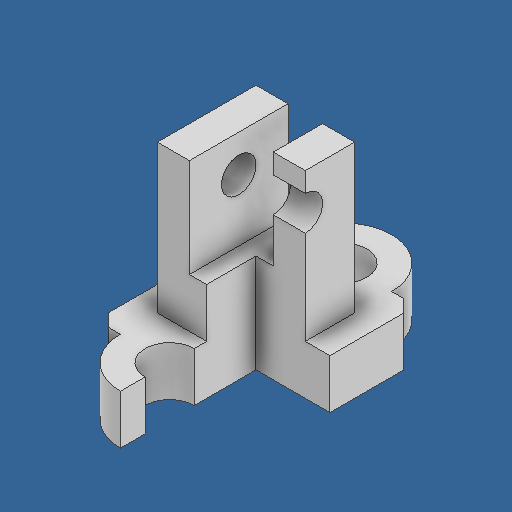
# Autodesk Inventor part: пч2020
Saved by Autodesk Inventor 2025 (Build 290162000, 162)
## iProperties
Created: 2024-12-02
Part Number: пч2020
Material: Типовые
Document SubType Name: Modeling
Designer: Asus
Density: 1 g/cm^3
Appearance: По умолчанию
Author: Asus
Autodesk Inventor part; units mm, degrees
ref_plane "YZ Plane" through (0, 0, 0) normal (1, 0, 0) x (0, 1, 0)
ref_plane "XY Plane" through (0, 0, 0) normal (0, 0, 1) x (1, 0, 0)
sketch "Эскиз1" plane through (0, 0, 0) normal (0, 1, 0) x (-1, 0, 0)
  line L0 (-30, 0) -> (-30, -30)
  line L1 (-30, 0) -> (-30, 30)
  circle A0 centre (0, 35) radius 10
  arc A1 (20, 35) -> (-20, 35) centre (0, 35) ccw
  line L2 (-25, 35) -> (-30, 30)
  circle A2 centre (0, -35) radius 10
  arc A3 (-20, -35) -> (20, -35) centre (0, -35) ccw
  line L3 (-30, -30) -> (-25, -35)
  line L4 (30, 30) -> (30, -30)
  line L5 (25, 35) -> (30, 30)
  line L6 (25, -35) -> (30, -30)
  line L7 (-25, 35) -> (-20, 35)
  line L8 (20, 35) -> (25, 35)
  line L9 (-25, -35) -> (-20, -35)
  line L10 (20, -35) -> (25, -35)
  point P0 (0, 0)
  point P1 (-30, -35)
  point P2 (-30, 35)
  point P3 (30, 35)
  point P4 (30, -35)
  point P5 (30, 35)
  point P6 (30, -35)
  dimension "d0" = 35
  dimension "d1" = 35
  dimension "d2" = 20
  dimension "d3" = 40
  dimension "d4" = 5
  dimension "d5" = 5
  dimension "d6" = 20
  dimension "d7" = 40
  dimension "d8" = 5
  dimension "d9" = 5
  dimension "d10" = 5
  dimension "d11" = 5
  dimension "d12" = 5
  dimension "d13" = 5
  constraints: 22 end point, 8 point on line, 4 centre point, 4 horizontal, 4 point on circle, 2 coincident, 2 perpendicular, 2 vertical
  measures "d0" distance of L0.start point (-30, -35)
  measures "d1" distance of L0.start point (-30, 35)
  measures "d2" diameter of A0
  measures "d3" diameter of A1
  measures "d4" distance of L2.start point (-30, 35)
  measures "d5" distance of L1.end point (-30, 35)
  measures "d6" diameter of A2
  measures "d7" diameter of A3
  measures "d8" distance of L0.end point (-30, -35)
  measures "d9" distance of L3.end point (-30, -35)
  measures "d10" distance of L5.start point (30, 35)
  measures "d11" distance of L4.start point (30, 35)
  measures "d12" distance of L6.start point (30, -35)
  measures "d13" distance of L4.end point (30, -35)
extrude "Выдавливание1" add sketch "Эскиз1" along normal blind 20
sketch "Эскиз2" plane through (0, 20, 0) normal (0, 1, 0) x (1, 0, 0)
  line L0 (20, 20) -> (-20, 20)
  line L1 (-20, 20) -> (-20, -20)
  line L2 (-20, -20) -> (20, -20)
  line L3 (20, -20) -> (20, 20)
  line L4 (20, 20) -> (-20, -20) construction
  line L5 (-20, 20) -> (20, -20) construction
  point P0 (0, 0)
  dimension "d16" = 40
  dimension "d17" = 40
  constraints: 12 end point, 2 midpoint, 2 parallel, 1 horizontal, 1 perpendicular
  measures "d16" distance of L2.end L1.end
  measures "d17" distance of L1.end L0.end
extrude "Выдавливание2" add sketch "Эскиз2" along normal blind 20
sketch "Эскиз3" plane through (0, 40, 0) normal (0, 1, 0) x (1, 0, 0)
  line L0 (-7, -20) -> (-7, 20)
  line L1 (-7, -20) -> (-20, -20)
  line L2 (-20, -20) -> (-20, 20)
  line L3 (7, -20) -> (7, 20)
  line L4 (20, -20) -> (7, -20)
  line L5 (-7, -20) -> (-20, -20)
  line L6 (-20, 20) -> (-7, 20)
  line L7 (20, 20) -> (20, -20) projected
  line L8 (20, -20) -> (20, 20)
  line L9 (20, 20) -> (7, 20)
  point P0 (0, 0)
  constraints: 18 end point, 1 horizontal, 1 perpendicular, 1 vertical
extrude "Выдавливание3" add sketch "Эскиз3" along normal blind 40
sketch "Эскиз4" plane through (20, 20, 20) normal (1, 0, 0) x (0, 0, -1)
  circle A0 centre (20, 45) radius 7
  point P0 (20, -20)
  dimension "d22" = 14
  constraints: 1 centre point
  measures "d22" diameter of A0
extrude "Выдавливание4" cut sketch "Эскиз4" against normal blind 40
ref_plane "РабПлоскость1" through (0, 80, 0) normal (0, 1, 0) x (-1, 0, 0)
sketch "Эскиз5" plane through (0, 80, 0) normal (0, 1, 0) x (-1, 0, 0)
  line L0 (0, 0) -> (-33, 0)
  line L1 (-33, 0) -> (-33, 61)
  line L2 (-33, 61) -> (0, 61)
  line L3 (0, 61) -> (0, 0)
  constraints: 8 end point, 2 parallel, 1 horizontal, 1 perpendicular
extrude "Выдавливание5" cut sketch "Эскиз5" against normal blind 80
equation "\"d5\" = d4"
equation "\"d9\" = d8"
equation "\"d11\" = d10"
equation "\"d12\" = d10"
equation "\"d13\" = d12"
